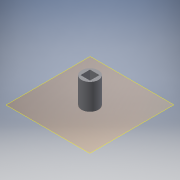
# Autodesk Inventor part: gear spacer 2
Saved by Autodesk Inventor 2017 (Build 210142000, 142)
## iProperties
Created: 2018-04-25
Part Number: gear spacer 2
Material: Generic
Document SubType Name: Modeling
Designer: RKL
Density: 1 g/cm^3
Appearance: Default
Author: RKL
Autodesk Inventor part; units mm, degrees
ref_plane "YZ Plane" through (0, 0, 0) normal (1, 0, 0) x (0, 1, 0)
ref_plane "XZ Plane" through (0, 0, 0) normal (0, 1, 0) x (-1, 0, 0)
ref_plane "Work Plane1" through (0, 0, 0) normal (0, 0, 1) x (1, 0, 0)
sketch "Sketch1" plane through (0, 0, 0) normal (0, 0, 1) x (1, 0, 0)
  line L0 (4.7625, 4.7625) -> (-4.7625, 4.7625) projected
  line L1 (-4.7625, 4.7625) -> (-4.7625, -4.7625) projected
  line L2 (-4.7625, -4.7625) -> (4.7625, -4.7625) projected
  line L3 (4.7625, -4.7625) -> (4.7625, 4.7625) projected
  circle A0 centre (0, 0) radius 8.5 projected
  point P0 (0, 0)
ref_plane "Work Plane2" through (-24.0297, -23.8955, 26) normal (0, 0, -1) x (0, 1, 0)
extrude "Extrusion1" add sketch "Sketch1" along normal up to surface (26 mm away)
body "Solid1"
